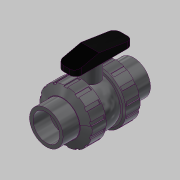
# Autodesk Inventor part: BALL VALVE MANUAL GLUED DN40
Saved by Autodesk Inventor 2017 (Build 210142000, 142)
## iProperties
Created: 2016-04-26
Part Number: BALL VALVE MANUAL GLUED DN40
Description: DUAL BLOCK VINK
Document SubType Name: Modeling
Manufacturer: SEKISUI
Mass: 197.859 g
Surface Area: 285.44 cm^2
Volume: 153.379 cm^3
Density: 1.29 g/cm^3
Material: U-PVC
Appearance: Smooth - Medium Gray
Title: BALL VALVE PVC-U TRD DN15
Autodesk Inventor part; units mm, degrees
ref_plane "YZ Plane" through (0, 0, 0) normal (1, 0, 0) x (0, 1, 0)
ref_plane "XZ Plane" through (0, 0, 0) normal (0, 1, 0) x (-1, 0, 0)
ref_plane "XY Plane" through (0, 0, 0) normal (0, 0, 1) x (1, 0, 0)
sketch "Sketch_1" plane through (0, 0, 0) normal (0, 0, 1) x (1, 0, 0)
  line L0 (51, 0) -> (51, -32.6667)
  line L1 (51, -32.6667) -> (45.0552, -49)
  line L2 (45.0552, -49) -> (18.5691, -49)
  line L3 (18.5691, -49) -> (17, -44.6888)
  line L4 (17, -44.6888) -> (17, -40.101)
  arc A0 (-17, -40.101) -> (17, -40.101) centre (0, 0) ccw
  line L5 (-17, -40.101) -> (-17, -44.6888)
  line L6 (-17, -44.6888) -> (-18.5691, -49)
  line L7 (-18.5691, -49) -> (-45.0552, -49)
  line L8 (-45.0552, -49) -> (-51, -32.6667)
  line L9 (-51, -32.6667) -> (-51, 0)
  line L10 (-51, 0) -> (51, 0)
  line L11 (-18.5691, -49) -> (0, -49) construction
  line L12 (0, -49) -> (0, -43.5556) construction
  line L13 (-45.7831, -49) -> (-20.5691, -49)
  line L14 (-20.5691, -49) -> (-20.5691, -47)
  line L15 (-20.5691, -47) -> (-45.7831, -47)
  line L16 (-45.7831, -47) -> (-45.7831, -49)
  line L17 (20.5691, -49) -> (45.7831, -49)
  line L18 (45.7831, -49) -> (45.7831, -47)
  line L19 (45.7831, -47) -> (20.5691, -47)
  line L20 (20.5691, -47) -> (20.5691, -49)
  point P0 (-31.8121, -49)
  dimension "dimZ" = 102
  dimension "dimE" = 98
  dimension "d22" = 49
  dimension "d23" = 16.3333
  dimension "d24" = 20
  dimension "d27" = 34
  dimension "d28" = 34
  dimension "d40" = 5.4444
  dimension "d52" = 20
  dimension "d53" = 2
  dimension "d54" = 2
  dimension "d55" = 2
  constraints: 42 end point, 6 parallel, 5 equal length, 5 perpendicular, 4 horizontal, 3 collinear, 3 point on circle, 3 point on line, 2 coincident, 2 midpoint, 1 centre point
  measures "dimZ" distance of L9.end L0.start
  measures "dimE" diameter of L2 L10
  measures "d22" distance from line of L0.start L2
  measures "d23" vertical distance of L0.end L1.end
  measures "d24" angle of L0 L1
  measures "d27" distance between parallel lines of L9 L5
  measures "d28" distance between parallel lines of L0 L4
  measures "d40" distance of L11.end L12.end
  measures "d52" angle of L5 L6
  measures "d53" distance of L15.end L13.start
  measures "d54" distance from line of L6.end L14
  measures "d55" distance from line of L2.end L20
revolve "Revolution1" add sketch "Sketch_1" angle 360 about axis through (-51, 0, 0) along (1, 0, 0) contours L0 L1 L19 L20 L2 L3 L4 A0 L5 L6 L7 L14 L15 L8 L9 L10 | L1 L2 L20 L19 | L15 L14 L7 L8
sketch "Sketch_2" plane through (0, 0, 0) normal (0, 0, 1) x (1, 0, 0)
  line L0 (0, 0) -> (0, 89)
  line L1 (0, 89) -> (17, 89)
  line L2 (17, 89) -> (17, 0)
  line L3 (17, 0) -> (0, 0)
  line L4 (0, 0) -> (0, 89)
  line L5 (17, -44.6888) -> (17, 44.6888) projected
  dimension "dimB" = 89
  constraints: 10 end point, 2 perpendicular, 1 coincident, 1 collinear, 1 vertical
  measures "dimB" distance of L0.start L0.end
revolve "Revolution2" add sketch "Sketch_2" angle 360 about axis through (0, 0, 0) along (0, -1, 0)
sketch "Sketch11" plane through (0, 89, 0) normal (0, 1, 0) x (1, 0, 0)
  circle A0 centre (0, 0) radius 17 projected
  line L0 (-44, 17) -> (64, 17)
  line L1 (64, 17) -> (64, -17)
  line L2 (64, -17) -> (-44, -17)
  line L3 (-44, -17) -> (-44, 17)
  dimension "dimC1" = 64
  dimension "dimC" = 108
  constraints: 8 end point, 2 parallel, 2 tangent, 1 horizontal, 1 perpendicular
  measures "dimC1" distance from line of L1 A0.centre
  measures "dimC" distance of L0.start L0.end
extrude "Extrusion6" add sketch "Sketch11" against normal blind 20 contours A0 L0 L1 L2 | A0 L2 L3 L0
fillet "Fillet1" radius 10.8 4 edges at (-44, 79, -17) (-44, 79, 17) (64, 79, 17) (64, 79, -17)
sketch "Sketch_7" plane through (0, 0, 0) normal (0, 0, 1) x (1, 0, 0)
  line L0 (-82, 31.5) -> (82, 31.5)
  line L1 (48.5126, 0) -> (-48.5126, 0)
  line L2 (-82, 31.5) -> (-82, 25)
  line L3 (-82, 25) -> (82, 25)
  line L4 (82, 25) -> (82, 31.5)
  line L5 (0, -4) -> (0, 24) projected
  point P0 (0, 0)
  point P1 (0, 0)
  point P2 (0, 25)
  dimension "dimH" = 164
  dimension "dimD" = 50
  dimension "dimD2" = 63
  constraints: 10 end point, 2 midpoint, 2 perpendicular, 1 coincident, 1 horizontal, 1 parallel, 1 point on line, 1 vertical
  measures "dimH" distance of L2.end L3.end
  measures "dimD" diameter of L3 L1
  measures "dimD2" diameter of L0 L1
revolve "Revolution3" add sketch "Sketch_7" angle 360 about axis through (48.5126, 0, 0) along (-1, 0, 0)
sketch "Sketch12" plane through (0, 0, 0) normal (0, 0, 1) x (1, 0, 0)
  line L0 (53.2, 89) -> (64, 89) projected
  line L1 (-33.2, 89) -> (53.2, 89) projected
  line L2 (-44, 89) -> (-33.2, 89) projected
  line L3 (-33.2, 89) -> (-44, 89) projected
  line L4 (53.2, 89) -> (-33.2, 89) projected
  line L5 (64, 89) -> (53.2, 89) projected
  line L6 (-44, 69) -> (-33.2, 69) projected
  line L7 (-33.2, 69) -> (-44, 69) projected
  line L8 (-33.2, 69) -> (0, 69) projected
  line L9 (0, 69) -> (0, 69) projected
  line L10 (0, 69) -> (-33.2, 69) projected
  line L11 (64, 69) -> (53.2, 69) projected
  line L12 (53.2, 69) -> (64, 69) projected
  line L13 (53.2, 69) -> (0, 69) projected
  line L14 (0, 69) -> (0, 69) projected
  line L15 (0, 69) -> (53.2, 69) projected
  line L16 (-44, 79) -> (-44, 89)
  line L17 (-44, 89) -> (0, 89)
  line L18 (0, 89) -> (-44, 79)
  line L19 (0, 89) -> (64, 89)
  line L20 (64, 89) -> (64, 79)
  line L21 (64, 79) -> (0, 89)
  line L22 (0, 0) -> (0, 89)
  point P0 (-58, 108)
  point P1 (-58, 84.5)
  point P2 (76, 84.5)
  dimension "d43" = 10
  dimension "d44" = 10
  dimension "d45" = 64
  dimension "d46" = 108
  constraints: 14 end point, 2 perpendicular, 2 point on line, 2 vertical, 1 collinear
  measures "d43" distance of L16.start L16.end
  measures "d44" distance of L19.end L20.end
  measures "d45" distance from line of L17.end L20
  measures "d46" distance between parallel lines of L20 L16
extrude "Extrusion7" cut sketch "Sketch12" along normal through all both and the other way through all
extrude "Extrusion8" cut sketch "Sketch_1" along normal mid plane 6.5333 contours L18 L17 L1 | L1 L2 L20 L19 | L15 L14 L7 L8 | L8 L13 L16
pattern_circular "Circular Pattern1" count 14 over 360 about axis through (41, 0, 0) along (-1, 0, 0) of "Extrusion8"
equation "\"d23\" = 0.333333 * d22"
equation "\"d27\" = 0.333333 * dimZ"
equation "\"d28\" = d27"
equation "\"d40\" = 0.333333 * d23"
equation "\"d33\" = 0.5 * dimB - 0.25 * dimE"
equation "\"d35\" = 0.1 * dimC"
equation "\"d43\" = 0.5 * d33"
equation "\"d44\" = 0.5 * d33"
equation "\"d45\" = dimC1"
equation "\"d46\" = dimC"
equation "\"d47\" = 0.0666667 * dimE"
equation "\"oMe\" = dimE"
body "Solid1"
